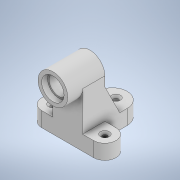
# Autodesk Inventor part: Крепление для дифферинциала
Saved by Autodesk Inventor 2020 (Build 240168000, 168)
## iProperties
Created: 2021-05-23
Part Number: Крепление для дифферинциала
Material: Типовые
Document SubType Name: Modeling
Designer: Антон
Density: 1 g/cm^3
Appearance: По умолчанию
Author: Антон
Autodesk Inventor part; units mm, degrees
ref_plane "YZ Plane" through (0, 0, 0) normal (1, 0, 0) x (0, 1, 0)
ref_plane "XZ Plane" through (0, 0, 0) normal (0, 1, 0) x (-1, 0, 0)
ref_plane "XY Plane" through (0, 0, 0) normal (0, 0, 1) x (1, 0, 0)
sketch "Эскиз1" plane through (0, 0, 0) normal (0, 0, 1) x (1, 0, 0)
  circle A0 centre (0, 0) radius 7.55
  circle A1 centre (0, 0) radius 10
  dimension "d0" = 15.1
  dimension "d1" = 20
  constraints: 2 centre point, 2 coincident
  measures "d0" diameter of A0
  measures "d1" diameter of A1
extrude "Выдавливание1" add sketch "Эскиз1" against normal blind 4
sketch "Эскиз2" plane through (0, 0, -4) normal (0, 0, -1) x (-1, 0, 0)
  circle A0 centre (0, 0) radius 10 projected
  circle A1 centre (0, 0) radius 7.55 projected
  circle A2 centre (0, 0) radius 6.5
  dimension "d4" = 13
  constraints: 1 centre point, 1 coincident
  measures "d4" diameter of A2
extrude "Выдавливание2" add sketch "Эскиз2" along normal blind 6 contours A0 | A1
sketch "Эскиз3" plane through (0, 0, -10) normal (0, 0, -1) x (-1, 0, 0)
  circle A0 centre (0, 0) radius 10 projected
  circle A1 centre (0, 0) radius 6.5 projected
  line L0 (-10, -6.5) -> (10, -6.5)
  line L1 (10, -6.5) -> (10, -36.5)
  line L2 (10, -36.5) -> (-10, -36.5)
  line L3 (-10, -36.5) -> (-10, -6.5)
  line L4 (-10, -6.5) -> (-10, 0)
  circle A2 centre (0, 0) radius 10 projected
  line L5 (10, -6.5) -> (10, 0)
  point P0 (0, -6.5)
  point P1 (-10, 0)
  dimension "d7" = 20
  dimension "d8" = 30
  constraints: 12 end point, 3 perpendicular, 2 parallel, 1 horizontal, 1 horizontal alignment, 1 midpoint, 1 tangent, 1 vertical alignment, 3 other
  measures "d7" distance of L1.end L2.end
  measures "d8" distance of L0.end L1.end
extrude "Выдавливание3" add sketch "Эскиз3" along normal blind 15
sketch "Эскиз4" plane through (-10, -36.5, -10) normal (0, -1, 0) x (1, 0, 0)
  line L0 (0, -15) -> (20, -15) projected
  line L1 (20, -15) -> (35, -15)
  line L2 (35, -15) -> (35, 0)
  line L3 (35, 0) -> (20, 0)
  line L4 (20, 0) -> (20, -15)
  line L5 (20, 0) -> (0, 0) projected
  point P0 (10, 10)
  constraints: 8 end point, 2 parallel, 2 perpendicular, 1 collinear, 1 horizontal
extrude "Выдавливание4" add sketch "Эскиз4" against normal blind 10
sketch "Эскиз5" plane through (-10, -26.5, -10) normal (0, 1, 0) x (1, 0, 0)
  line L0 (35, 0) -> (35, 15) projected
  line L1 (35, 7.5) -> (20, 7.5)
  line L2 (20, 0) -> (20, 15) projected
  point P0 (10, -10)
  point P1 (27.5, 7.5)
  constraints: 3 midpoint, 2 end point
hole "Отверстие1" at (17.5, -26.5, -17.5) direction (0, -1, 0) diameter 3.2 end through all countersink diameter 6 countersink angle 90
fillet "Сопряжение1" radius 7.5 2 edges at (25, -31.5, -25) (25, -31.5, -10)
ref_plane "РабПлоскость1" through (0, -36.5, -10) normal (-1, 0, 0) x (0, 0, 1)
mirror "Зеркальное отражение1" about plane through (0, -36.5, -10) normal (-1, 0, 0) of "Отверстие1", "Сопряжение1", "Выдавливание4"
sketch "Эскиз6" plane through (0, 0, -25) normal (0, 0, -1) x (-1, 0, 0)
  line L0 (17.5, -36.5) -> (-17.5, -36.5) projected
  line L1 (-10, -6.5) -> (10, -6.5)
  line L2 (10, -6.5) -> (10, -36.5)
  line L3 (10, -36.5) -> (-10, -36.5)
  line L4 (-10, -36.5) -> (-10, -6.5)
  circle A0 centre (0, 0) radius 6.5 projected
  line L5 (10, -26.5) -> (10, 0) projected
  line L6 (-10, 0) -> (-10, -26.5) projected
  constraints: 8 end point, 2 collinear, 2 parallel, 1 horizontal, 1 perpendicular, 1 point on line, 1 tangent
extrude "Выдавливание5" add sketch "Эскиз6" along normal blind 10 contours L0 L4 L1 L2
sketch "Эскиз7" plane through (0, 0, -35) normal (0, 0, -1) x (-1, 0, 0)
  line L0 (-10, -6.5) -> (-10, -36.5) projected
  line L1 (10, -26.5) -> (10, 0) projected
  line L2 (-10, -36.5) -> (10, -36.5)
  line L3 (10, -36.5) -> (10, -26.5)
  line L4 (10, -26.5) -> (-10, -26.5)
  line L5 (-10, -26.5) -> (-10, -36.5)
  point P0 (0, 0)
  constraints: 8 end point, 2 parallel, 1 horizontal, 1 perpendicular
extrude "Выдавливание6" add sketch "Эскиз7" along normal blind 15
sketch "Эскиз8" plane through (-10, -26.5, -35) normal (0, 1, 0) x (1, 0, 0)
  line L0 (0, 15) -> (20, 15) projected
  line L1 (10, 15) -> (10, 0)
  line L2 (20, 0) -> (0, 0) projected
  point P0 (10, -35)
  point P1 (10, 7.5)
  constraints: 3 midpoint, 2 end point
hole "Отверстие2" at (0, -26.5, -42.5) direction (0, -1, 0) diameter 3.2 end through all countersink diameter 6 countersink angle 90
fillet "Сопряжение2" radius 10 2 edges at (10, -31.5, -50) (-10, -31.5, -50)
chamfer "Фаска1" distance 20 distance2 10 1 edges at (0, -6.5, -35) measured on face at (0, -7, -35)
